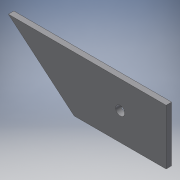
# Autodesk Inventor part: mount2
Saved by Autodesk Inventor 2018.2 (Build 222227000, 227)
## iProperties
Created: 2018-04-27
Part Number: mount2
Material: 一般
Document SubType Name: Modeling
Designer: ku_sk
Density: 1 g/cm^3
Appearance: 既定
Author: ku_sk
Autodesk Inventor part; units mm, degrees
ref_plane "YZ Plane" through (0, 0, 0) normal (1, 0, 0) x (0, 1, 0)
ref_plane "XZ Plane" through (0, 0, 0) normal (0, 1, 0) x (-1, 0, 0)
ref_plane "XY Plane" through (0, 0, 0) normal (0, 0, 1) x (1, 0, 0)
sketch "スケッチ1" plane through (0, 0, 0) normal (0, 1, 0) x (-1, 0, 0)
  circle A0 centre (0, 0) radius 2.5
  line L0 (-25, 15) -> (60.7526, 15)
  line L1 (-25, -15) -> (-25, 15)
  line L2 (-25, -15) -> (25, -15)
  line L3 (25, -15) -> (60.7526, 15)
  line L4 (0, -21) -> (0, 21) projected
  line L5 (77.9031, 0) -> (-42.1505, 0) projected
  dimension "d0" = 5
  dimension "d3" = 15
  dimension "d4" = 15
  dimension "d5" = 25
  dimension "d6" = 40
  dimension "d7" = 50
  constraints: 8 end point, 2 parallel, 1 centre point, 1 coincident, 1 horizontal
  measures "d0" diameter of A0
  measures "d3" distance from line of point (0, 0) L0
  measures "d4" distance from line of L2 point (0, 0)
  measures "d5" distance from line of point (0, 0) L1
  measures "d6" angle of L2 L3
  measures "d7" distance of L1.start L2.end
extrude "押し出し1" add sketch "スケッチ1" along normal mid plane 3 contours L5 L3 L2 L4 A0 | A0 L4 L0 L3 L5 | A0 L5 L1 L0 L4 | L4 L2 L1 L5 A0
equation "\"d4\" = d3"
